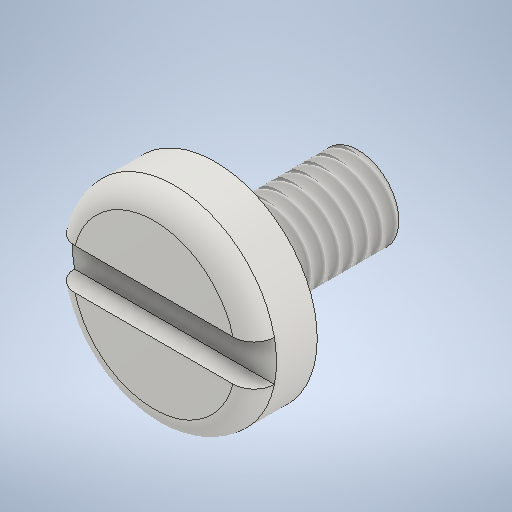
# Autodesk Inventor part: 17A - Crosshead pin1
Saved by Autodesk Inventor 2025.2 (Build 292293000, 293)
## iProperties
Created: 2025-06-19
Part Number: 17A - Crosshead pin1
Material: Steel AISI 1020 107 HR
Document SubType Name: Modeling
Designer: bless
Density: 7.87 g/cm^3
Appearance: Steel
Author: bless
Autodesk Inventor part; units mm, degrees
ref_plane "YZ Plane" through (0, 0, 0) normal (1, 0, 0) x (0, 1, 0)
ref_plane "XZ Plane" through (0, 0, 0) normal (0, 1, 0) x (-1, 0, 0)
ref_plane "XY Plane" through (0, 0, 0) normal (0, 0, 1) x (1, 0, 0)
sketch "Sketch1" plane through (0, 0, 0) normal (0, 0, 1) x (1, 0, 0)
  circle A0 centre (0, 0) radius 5
  dimension "d0" = 10
  constraints: 1 centre point, 1 coincident
  measures "d0" diameter of A0
extrude "Extrusion1" add sketch "Sketch1" along normal blind 3
sketch "Sketch2" plane through (0, 0, 3) normal (0, 0, 1) x (1, 0, 0)
  circle A0 centre (0, 0) radius 5 projected
  line L0 (-4.899, 1) -> (4.899, 1)
  line L1 (7.3763, 1) -> (7.3763, -1)
  line L2 (4.899, -1) -> (-4.899, -1)
  line L3 (-7.3763, -1) -> (-7.3763, 1)
  line L4 (-7.3763, 1) -> (7.3763, -1) construction
  line L5 (7.3763, 1) -> (-7.3763, -1) construction
  circle A1 centre (0, 0) radius 5 projected
  dimension "d3" = 2
  dimension "d4" = 82.28
  dimension "d5" = 82.28
  dimension "d6" = 2
  dimension "d7" = 1
  constraints: 12 end point, 4 point on circle, 2 midpoint, 2 parallel, 1 horizontal, 1 perpendicular
  measures "d3" distance of L3.start L3.end
  measures "d4" angle of L1 L5
  measures "d5" angle of L1 L4
  measures "d6" distance between parallel lines of L0 L2
  measures "d7" distance from line of A0.centre L0
extrude "Extrusion2" cut sketch "Sketch2" against normal blind 1 contours A0 L2 L0
fillet "Fillet1" radius 1 2 edges at (0, 5, 3) (0, -5, 3)
sketch "Sketch3" plane through (0, 0, 0) normal (0, 0, -1) x (-1, 0, 0)
  circle A0 centre (0, 0) radius 5 projected
  circle A1 centre (0, 0) radius 2
  dimension "d11" = 4
  constraints: 1 centre point, 1 coincident
  measures "d11" diameter of A1
extrude "Extrusion3" add sketch "Sketch3" along normal blind 7 contours A1
thread "Thread1" size "M4x0.7" class "6g" standard "ANSI Metric M Profile" length 7
body "Solid1"
